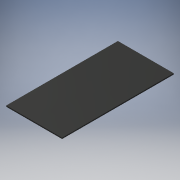
# Autodesk Inventor part: chapa de metal
Saved by Autodesk Inventor 2018 (Build 220112000, 112)
## iProperties
Created: 2018-09-22
Part Number: chapa de metal
Material: Aço
Document SubType Name: Chapa de metal
Designer: Usuario
Density: 7.85 g/cm^3
Sheet Metal Rule: Padrão_mm
Appearance: Placa
Author: Usuario
Autodesk Inventor part; units mm, degrees
ref_plane "YZ Plane" through (0, 0, 0) normal (1, 0, 0) x (0, 1, 0)
ref_plane "XZ Plane" through (0, 0, 0) normal (0, 1, 0) x (-1, 0, 0)
ref_plane "XY Plane" through (0, 0, 0) normal (0, 0, 1) x (1, 0, 0)
sketch "Esboço1" plane through (0, 0, 0) normal (0, 0, 1) x (1, 0, 0)
  line L0 (-75, 150) -> (75, 150)
  line L1 (75, 150) -> (75, -150)
  line L2 (75, -150) -> (-75, -150)
  line L3 (-75, -150) -> (-75, 150)
  line L4 (-75, 150) -> (75, -150) construction
  line L5 (75, 150) -> (-75, -150) construction
  point P0 (0, 0)
  dimension "d0" = 300
  dimension "d1" = 150
  measures "d0" distance of L0.end L1.end
  measures "d1" distance of L1.end L2.end
extrude "Placa1" add sketch "Esboço1" along normal blind 3
equation "\"d2\" = Espessura"
equation "\"Raio_vergadura\" = Espessura"
equation "\"Largura_alívio_de_vergadura\" = Espessura"
equation "\"Profundidade_alívio_de_vergadura\" = 0.5 * Espessura"
equation "\"Tamanho_alívio_de_dobra\" = 4 * Espessura"
equation "\"Remanescente_mínimo\" = 2 * Espessura"
equation "\"Raiodetransição\" = Raio_vergadura"
equation "\"Tamanho_de_raio_de_Jacobi\" = Raio_vergadura"
equation "\"TamanhoFolga\" = Espessura"
equation "\"Espessura\" = 3"
